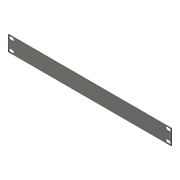
# Autodesk Inventor part: PatchPanel_front
Saved by Autodesk Inventor 2017 (Build 210142000, 142)
## iProperties
Created: 2018-03-19
Part Number: PatchPanel_front
Material: Generic
Document SubType Name: Modeling
Designer: Kathryn Rosie
Density: 1 g/cm^3
Appearance: Galvanized
Author: Kathryn Rosie
Autodesk Inventor part; units mm, degrees
ref_plane "YZ Plane" through (0, 0, 0) normal (1, 0, 0) x (0, 1, 0)
ref_plane "XZ Plane" through (0, 0, 0) normal (0, 1, 0) x (-1, 0, 0)
ref_plane "XY Plane" through (0, 0, 0) normal (0, 0, 1) x (1, 0, 0)
sketch "Sketch1" plane through (0, 0, 0) normal (0, 0, 1) x (1, 0, 0)
  line L0 (-241.3, -22.225) -> (241.3, -22.225)
  line L1 (241.3, -22.225) -> (241.3, 22.225)
  line L2 (241.3, 22.225) -> (-241.3, 22.225)
  line L3 (-241.3, 22.225) -> (-241.3, -22.225)
  line L4 (-241.3, -22.225) -> (241.3, 22.225) construction
  line L5 (241.3, -22.225) -> (-241.3, 22.225) construction
  point P0 (0, 0)
  dimension "d0" = 482.6
  dimension "d1" = 44.45
  constraints: 12 end point, 2 midpoint, 2 parallel, 1 horizontal, 1 perpendicular
  measures "d0" distance of L2.end L1.end
  measures "d1" distance of L2.end L0.start
extrude "Extrusion1" add sketch "Sketch1" along normal blind 2
sketch "Sketch2" plane through (0, 0, 2) normal (0, 0, 1) x (1, 0, 0)
  line L0 (-235.2675, 15.875) -> (-228.9175, 15.875) construction
  line L1 (-235.2675, 10.875) -> (-228.9175, 10.875)
  line L2 (-228.9175, 20.875) -> (-235.2675, 20.875)
  arc A0 (-235.2675, 20.875) -> (-235.2675, 10.875) centre (-235.2675, 15.875) ccw
  arc A1 (-228.9175, 10.875) -> (-228.9175, 20.875) centre (-228.9175, 15.875) ccw
  line L3 (241.3, 22.225) -> (-241.3, 22.225) projected
  line L4 (-241.3, 22.225) -> (-241.3, -22.225) projected
  line L5 (-241.3, 0) -> (241.3, 0) construction
  line L6 (0, 22.225) -> (0, -22.225) construction
  line L7 (-235.2675, -15.875) -> (-228.9175, -15.875) construction
  line L8 (-235.2675, -10.875) -> (-228.9175, -10.875)
  line L9 (-228.9175, -20.875) -> (-235.2675, -20.875)
  arc A2 (-235.2675, -10.875) -> (-235.2675, -20.875) centre (-235.2675, -15.875) ccw
  arc A3 (-228.9175, -20.875) -> (-228.9175, -10.875) centre (-228.9175, -15.875) ccw
  line L10 (235.2675, 15.875) -> (228.9175, 15.875) construction
  line L11 (235.2675, 10.875) -> (228.9175, 10.875)
  line L12 (228.9175, 20.875) -> (235.2675, 20.875)
  arc A4 (235.2675, 10.875) -> (235.2675, 20.875) centre (235.2675, 15.875) ccw
  arc A5 (228.9175, 20.875) -> (228.9175, 10.875) centre (228.9175, 15.875) ccw
  line L13 (235.2675, -15.875) -> (228.9175, -15.875) construction
  line L14 (235.2675, -10.875) -> (228.9175, -10.875)
  line L15 (228.9175, -20.875) -> (235.2675, -20.875)
  arc A6 (235.2675, -20.875) -> (235.2675, -10.875) centre (235.2675, -15.875) ccw
  arc A7 (228.9175, -10.875) -> (228.9175, -20.875) centre (228.9175, -15.875) ccw
  point P0 (0, 0)
  point P1 (-232.0925, 15.875)
  point P2 (-232.0925, -15.875)
  point P3 (232.0925, 15.875)
  point P4 (232.0925, -15.875)
  dimension "d13" = 5
  dimension "d14" = 6.35
  dimension "d15" = 6.35
  dimension "d16" = 9.2075
  constraints: 36 end point, 21 symmetric about line, 16 point on circle, 8 centre point, 4 tangent, 3 midpoint, 2 horizontal, 1 parallel, 1 vertical, 6 other
  measures "d13" radius of A1
  measures "d14" distance of L2.start L2.end
  measures "d15" distance from line of point (-232.092, 15.875) L3
  measures "d16" distance from line of point (-232.092, 15.875) L4
extrude "Extrusion2" cut sketch "Sketch2" against normal up to surface (2 mm away)
body "Solid1"
